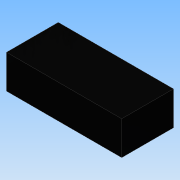
# Autodesk Inventor part: LCD Reader INCOMPLETE
Saved by Autodesk Inventor 2015 (Build 190159000, 159)
## iProperties
Created: 2014-11-11
Part Number: LCD Reader INCOMPLETE
Material: Generic
Document SubType Name: Modeling
Designer: 0
Density: 1 g/cm^3
Appearance: Default
Author: 0
Autodesk Inventor part; units mm, degrees
ref_plane "YZ Plane" through (0, 0, 0) normal (1, 0, 0) x (0, 1, 0)
ref_plane "XZ Plane" through (0, 0, 0) normal (0, 1, 0) x (-1, 0, 0)
ref_plane "XY Plane" through (0, 0, 0) normal (0, 0, 1) x (1, 0, 0)
sketch "Sketch1" plane through (0, 0, 0) normal (0, 1, 0) x (-1, 0, 0)
  line L0 (0, 0) -> (90.424, 0)
  line L1 (90.424, 0) -> (90.424, -40.64)
  line L2 (90.424, -40.64) -> (0, -40.64)
  line L3 (0, -40.64) -> (0, 0)
  dimension "d0" = 90.424
  dimension "d1" = 40.64
  constraints: 8 end point, 2 parallel, 1 horizontal, 1 perpendicular
  measures "d0" distance of L1.end L2.end
  measures "d1" distance of L0.end L1.end
extrude "Extrusion1" add sketch "Sketch1" along normal blind 26.416
body "Solid1"
